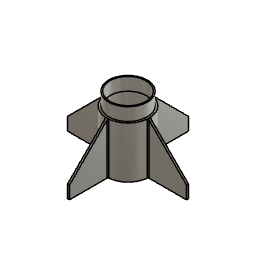
Fin Assembly v1 (Autodesk Fusion 360 design; units mm, degrees)
Autodesk Fusion 360 part; units mm, degrees
sketch "Sketch1" plane through (0, 0, 0) normal (0, 1, 0) x (1, 0, 0)
  circle A0 centre (0, 0) radius 38.1
  line L0 (0, 118.11) -> (1.905, 118.11)
  line L1 (0, 118.11) -> (-1.905, 118.11)
  line L2 (-1.905, 118.11) -> (-1.905, 41.8667)
  line L3 (1.905, 118.11) -> (1.905, 41.8667)
  line L4 (-118.11, -1.905) -> (-41.8667, -1.905)
  line L5 (-118.11, 1.905) -> (-41.8667, 1.905)
  line L6 (-118.11, 0) -> (-118.11, 1.905)
  line L7 (-118.11, 0) -> (-118.11, -1.905)
  line L8 (1.905, -118.11) -> (1.905, -41.8667)
  line L9 (-1.905, -118.11) -> (-1.905, -41.8667)
  line L10 (0, -118.11) -> (-1.905, -118.11)
  line L11 (0, -118.11) -> (1.905, -118.11)
  line L12 (118.11, 1.905) -> (41.8667, 1.905)
  line L13 (118.11, -1.905) -> (41.8667, -1.905)
  line L14 (118.11, 0) -> (118.11, -1.905)
  line L15 (118.11, 0) -> (118.11, 1.905)
  arc A1 (41.8667, 1.905) -> (1.905, 41.8667) centre (0, 0) ccw
  arc A2 (-1.905, 41.8667) -> (-41.8667, 1.905) centre (0, 0) ccw
  arc A3 (-41.8667, -1.905) -> (-1.905, -41.8667) centre (0, 0) ccw
  arc A4 (1.905, -41.8667) -> (41.8667, -1.905) centre (0, 0) ccw
  dimension "d3" = 1.905
  dimension "d4" = 1.905
  dimension "d6" = 360
  constraint coincident A0.centre A1.centre
  constraint horizontal L0
  constraint horizontal L1
  constraint perpendicular L1 L2
  constraint perpendicular L1 L3
  constraint concentric A0 A2
  constraint concentric A1 A2
  constraint concentric A2 A3
  constraint concentric A3 A4
  measures "d3" distance of L0.start L0.end
  measures "d4" distance of L0.start L1.end
extrude "Extrude1" add sketch "Sketch1" along normal blind 101.6 makes body 1
chamfer "Chamfer1" distance 76.2 angle 45 4 edges at (118.11, 101.6, 0) (0, 101.6, 118.11) (-118.11, 101.6, 0) (0, 101.6, -118.11) on bodies 1
sketch "Sketch2" plane through (0, 101.6, 0) normal (0, 1, 0) x (-1, 0, 0)
  circle A0 centre (0, 0) radius 38.1
  line L0 (-1.905, -41.91) -> (1.905, -41.91)
  line L1 (1.905, -41.91) -> (1.905, -41.8667)
  arc A1 (1.905, -41.8667) -> (41.8667, -1.905) centre (0, 0) ccw
  line L2 (41.8667, -1.905) -> (41.91, -1.905)
  line L3 (41.91, -1.905) -> (41.91, 1.905)
  line L4 (41.91, 1.905) -> (41.8667, 1.905)
  arc A2 (41.8667, 1.905) -> (1.905, 41.8667) centre (0, 0) ccw
  line L5 (1.905, 41.8667) -> (1.905, 41.91)
  line L6 (1.905, 41.91) -> (-1.905, 41.91)
  line L7 (-1.905, 41.91) -> (-1.905, 41.8667)
  arc A3 (-1.905, 41.8667) -> (-41.8667, 1.905) centre (0, 0) ccw
  line L8 (-41.8667, 1.905) -> (-41.91, 1.905)
  line L9 (-41.91, 1.905) -> (-41.91, -1.905)
  line L10 (-41.91, -1.905) -> (-41.8667, -1.905)
  arc A4 (-41.8667, -1.905) -> (-1.905, -41.8667) centre (0, 0) ccw
  line L11 (-1.905, -41.8667) -> (-1.905, -41.91)
  circle A5 centre (0, 0) radius 35.56
  dimension "d11" = -2.54
extrude "Extrude2" add sketch "Sketch2" along normal blind 25.4 separate body contours A0 makes body 2
fillet "Fillet1" radius 1.905 7 edges at (1.905, 50.8, 41.8667) (41.8667, 50.8, 1.905) (41.8667, 50.8, -1.905) (1.905, 50.8, -41.8667) (-1.905, 50.8, -41.8667) (-41.8667, 50.8, -1.905) (-41.8667, 50.8, 1.905) on bodies 1
fillet "Fillet2" radius 1.905 1 edges at (-1.905, 50.8, 41.8667) on bodies 1
